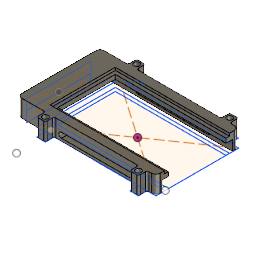
Mounting_plate_96_v3 v7 (Autodesk Fusion 360 design; units mm, degrees)
Autodesk Fusion 360 part; units mm, degrees
note: some values were not read from the file. Set by a fixed rule: which sketch regions a step uses.
sketch "Sketch1" plane through (0, 0, 0) normal (0, 0, 1) x (1, 0, 0)
  line L0 (-68.38, 47.37) -> (68.38, 47.37)
  line L1 (68.38, 47.37) -> (68.38, -47.37)
  line L2 (68.38, -47.37) -> (-68.38, -47.37)
  line L3 (-68.38, -47.37) -> (-68.38, 47.37)
  line L4 (-68.38, 47.37) -> (68.38, -47.37) construction
  line L5 (68.38, 47.37) -> (-68.38, -47.37) construction
  line L6 (-58.38, 57.37) -> (-48.38, 57.37)
  line L7 (-48.38, 57.37) -> (-48.38, 47.37)
  line L8 (-48.38, 47.37) -> (-58.38, 47.37)
  line L9 (-58.38, 47.37) -> (-58.38, 57.37)
  line L10 (48.38, 57.37) -> (58.38, 57.37)
  line L11 (58.38, 57.37) -> (58.38, 47.37)
  line L12 (58.38, 47.37) -> (48.38, 47.37)
  line L13 (48.38, 47.37) -> (48.38, 57.37)
  line L14 (48.38, -47.37) -> (58.38, -47.37)
  line L15 (58.38, -47.37) -> (58.38, -57.37)
  line L16 (58.38, -57.37) -> (48.38, -57.37)
  line L17 (48.38, -57.37) -> (48.38, -47.37)
  line L18 (-58.38, -47.37) -> (-48.38, -47.37)
  line L19 (-48.38, -47.37) -> (-48.38, -57.37)
  line L20 (-48.38, -57.37) -> (-58.38, -57.37)
  line L21 (-58.38, -57.37) -> (-58.38, -47.37)
  line L22 (68.38, 47.37) -> (68.38, 37)
  line L23 (68.38, -47.37) -> (68.38, -36.63)
  line L24 (68.38, 37) -> (-62.58, 37)
  line L25 (-62.58, 37) -> (-62.58, -37)
  line L26 (-62.58, -37) -> (68.38, -37)
  line L27 (68.38, -37) -> (68.38, 37)
  line L28 (68.38, 37) -> (68.38, 33)
  line L29 (68.38, 33) -> (-58.58, 33)
  line L30 (-58.58, 33) -> (-58.58, -33)
  line L31 (-58.58, -33) -> (68.38, -33)
  line L32 (68.38, -33) -> (68.38, 33)
  point P0 (-57.3369, -42.2056)
  point P1 (-53.88, -84.89)
  dimension "d1" = 136.76
  dimension "d2" = 94.74
  dimension "d3" = 10
  dimension "d4" = 10
  dimension "d5" = 10
  dimension "d6" = 10
  dimension "d15" = 10.37
  dimension "d16" = 10.74
  dimension "d17" = 74
  dimension "d18" = 130.96
  dimension "d19" = 4
  dimension "d20" = 66
  dimension "d21" = 126.96
  constraint perpendicular L0 L1
  constraint parallel L0 L2
  constraint parallel L1 L3
  constraint horizontal L0
  constraint horizontal L6
  constraint vertical L7
  constraint horizontal L8
  constraint vertical L9
  constraint coincident L0 L7.end
  constraint horizontal L10
  constraint vertical L11
  constraint horizontal L12
  constraint vertical L13
  constraint horizontal L14
  constraint vertical L15
  constraint horizontal L16
  constraint vertical L17
  constraint horizontal L18
  constraint vertical L19
  constraint horizontal L20
  constraint vertical L21
  constraint perpendicular L0 L22
  constraint perpendicular L2 L23
  constraint horizontal L24
  constraint vertical L25
  constraint horizontal L26
  constraint vertical L27
  constraint perpendicular L24 L28
  constraint horizontal L29
  constraint vertical L30
  constraint horizontal L31
  constraint vertical L32
  measures "d1" distance of L1 L3
  measures "d2" distance of L0.start L2.end
  measures "d3" distance of L6.start L6.end
  measures "d4" distance of L6.start L8.end
  measures "d5" distance of L10.start L10.end
  measures "d6" distance of L10.start L12.end
  measures "d15" distance of L0.end L22.end
  measures "d16" distance of L1.end L23.end
  measures "d17" distance of L22.end L26.end
  measures "d18" distance of L22.end L24.end
  measures "d19" distance of L22.end L28.end
  measures "d20" distance of L28.end L31.end
  measures "d21" distance of L28.end L29.end
  measures "d160" distance of L0.end
extrude "Extrude2" add sketch "Sketch1" along normal blind 20 contours L0 L1 L2 L3 L8 L12 L14 L18 L22 L23 L24 L25 L26 | L0 L6 L7 L8 L9 | L2 L18 L19 L20 L21 | L0 L10 L11 L12 L13 | L2 L14 L15 L16 L17 | L1 L23 L24 L25 L26 L27 L28 L29 L30 L31
ref_plane "WorkPlane2" through (0, 0, 20) normal (0, 0, 1) x (1, 0, 0)
sketch "Sketch4" plane through (0, 0, 20) normal (0, 0, 1) x (1, 0, 0)
  line L0 (68.38, 37) -> (-62.58, 37)
  line L1 (-62.58, 37) -> (-62.58, -37.7)
  line L2 (-62.58, -37.7) -> (68.38, -37.7)
  line L3 (68.38, -37.7) -> (68.38, 37)
  dimension "d30" = 130.96
  dimension "d31" = 74.7
  constraint horizontal L0
  constraint vertical L1
  constraint horizontal L2
  constraint vertical L3
  measures "d30" distance of L0.start L0.end
  measures "d31" distance of L0.start L2.end
extrude "Extrude3" cut sketch "Sketch4" against normal blind 3
ref_plane "WorkPlane3" through (0, 0, 20) normal (0, 0, 1) x (1, 0, 0)
sketch "Sketch5" plane through (0, 0, 20) normal (0, 0, 1) x (1, 0, 0)
  circle A0 centre (-53.38, 52.37) radius 3.25
  circle A1 centre (53.38, 52.37) radius 3.25
  circle A2 centre (-53.38, -52.37) radius 3.25
  circle A3 centre (53.38, -52.37) radius 3.25
  dimension "d35" = 6.5
  dimension "d38" = 106.76
  dimension "d39" = -104.74
  measures "d35" diameter of A0
extrude "Extrude4" cut sketch "Sketch5" against normal blind 20
ref_plane "WorkPlane5" through (68.38, 0, 0) normal (1, 0, 0) x (0, 1, 0)
ref_plane "WorkPlane6" through (68.38, 0, 0) normal (1, 0, 0) x (0, 1, 0)
sketch "Sketch7" plane through (68.38, 0, 0) normal (1, 0, 0) x (0, 1, 0)
  line L0 (40.5, 12) -> (-40.5, 12)
  line L1 (-40.5, 12) -> (-40.5, -12)
  line L2 (-40.5, -12) -> (40.5, -12)
  line L3 (40.5, -12) -> (40.5, 12)
  line L4 (40.5, 12) -> (-40.5, -12) construction
  line L5 (-40.5, 12) -> (40.5, -12) construction
  dimension "d45" = 81
  dimension "d46" = 24
  constraint perpendicular L0 L1
  constraint parallel L0 L2
  constraint parallel L1 L3
  constraint horizontal L0
  constraint coincident L4 origin
  constraint coincident L5 origin
  measures "d45" distance of L1.end L2.end
  measures "d46" distance of L0.end L1.end
extrude "Extrude5" cut sketch "Sketch7" against normal blind 136.76
fillet "Fillet2" radius 2 16 edges at (-58.38, 57.37, 10) (-58.38, 47.37, 10) (-58.38, -47.37, 10) (-58.38, -57.37, 10) (-48.38, -57.37, 10) (-48.38, -47.37, 10) (58.38, -57.37, 10) (58.38, -47.37, 10) (48.38, -47.37, 10) (48.38, -57.37, 10) (58.38, 47.37, 10) (58.38, 57.37, 10) (48.38, 47.37, 10) (48.38, 57.37, 10) (-48.38, 47.37, 10) (-48.38, 57.37, 10)
ref_plane "WorkPlane7" through (0, -47.37, 10) normal (0, -1, 0) x (1, 0, 0)
delete_face "DeleteFace1" 1 faces at (15.46, -47.37, 6.6667)
ref_plane "WorkPlane9" through (0, -47.37, 10) normal (0, -1, 0) x (1, 0, 0)
sketch "Sketch10" plane through (0, -47.37, 10) normal (0, -1, 0) x (1, 0, 0)
  line L0 (0, -10) -> (0, -4)
  line L1 (40, -7) -> (-40, -7)
  line L2 (-40, -7) -> (-40, -1)
  line L3 (-40, -1) -> (40, -1)
  line L4 (40, -1) -> (40, -7)
  line L5 (40, -7) -> (-40, -1) construction
  line L6 (-40, -7) -> (40, -1) construction
  circle A0 centre (-40, -4) radius 3
  circle A1 centre (40, -4) radius 3
  point P0 (0, -4)
  dimension "d72" = 6
  dimension "d73" = 6
  dimension "d74" = 80
  dimension "d75" = 6
  dimension "d76" = 6
  constraint vertical L0
  constraint perpendicular L1 L2
  constraint parallel L1 L3
  constraint parallel L2 L4
  constraint horizontal L1
  constraint coincident L5 P0
  constraint coincident L6 P0
  constraint coincident P0 L0.end
  constraint midpoint L2 A0.centre
  constraint midpoint L4 A1.centre
  measures "d72" distance of L0.start P0
  measures "d73" distance of L1.end L2.end
  measures "d74" distance of L2.end L3.end
  measures "d75" diameter of A0
  measures "d76" diameter of A1
extrude "Extrude9" cut sketch "Sketch10" against normal blind 6.87
ref_plane "WorkPlane10" through (0, 47.37, 10) normal (0, 1, 0) x (-1, 0, 0)
sketch "Sketch11" plane through (0, 47.37, 10) normal (0, 1, 0) x (1, 0, 0)
  line L0 (0, 10) -> (0, 4)
  line L1 (-40, 7) -> (40, 7)
  line L2 (40, 7) -> (40, 1)
  line L3 (40, 1) -> (-40, 1)
  line L4 (-40, 1) -> (-40, 7)
  line L5 (-40, 7) -> (40, 1) construction
  line L6 (40, 7) -> (-40, 1) construction
  circle A0 centre (40, 4) radius 3
  circle A1 centre (-40, 4) radius 3
  point P0 (0, 4)
  dimension "d80" = 6
  dimension "d81" = 80
  dimension "d82" = 6
  dimension "d83" = 6
  dimension "d84" = 6
  constraint vertical L0
  constraint perpendicular L1 L2
  constraint parallel L1 L3
  constraint parallel L2 L4
  constraint horizontal L1
  constraint coincident L5 P0
  constraint coincident L6 P0
  constraint coincident P0 L0.end
  constraint midpoint L2 A0.centre
  constraint midpoint L4 A1.centre
  measures "d80" distance of L0.start P0
  measures "d81" distance of L2.end L3.end
  measures "d82" distance of L1.end L2.end
  measures "d83" diameter of A0
  measures "d84" diameter of A1
extrude "Extrude10" cut sketch "Sketch11" against normal blind 6.87
ref_plane "WorkPlane11" through (0, 0, 0) normal (0, 0, 1) x (1, 0, 0)
sketch "Sketch12" plane through (0, 0, 0) normal (0, 0, 1) x (1, 0, 0)
ref_plane "WorkPlane12" through (-68.38, 0, 10) normal (-1, 0, 0) x (0, -1, 0)
ref_plane "WorkPlane13" through (-68.38, 0, 10) normal (-1, 0, 0) x (0, -1, 0)
sketch "Sketch19" plane through (68.38, 0, 0) normal (1, 0, 0) x (0, 1, 0)
ref_plane "WorkPlane19" through (-68.38, 0, 10) normal (-1, 0, 0) x (0, -1, 0)
sketch "Sketch21" plane through (-68.38, 0, 10) normal (-1, 0, 0) x (0, 1, 0)
  line L0 (42, -2) -> (-42, -2)
  line L1 (42, -2) -> (-42, 22) construction
  line L2 (-42, -2) -> (42, 22) construction
  line L3 (42, -2) -> (-42, -2)
  line L4 (-42, -2) -> (-42, 10)
  line L5 (-42, 10) -> (42, 10)
  line L6 (42, 10) -> (42, -2)
  point P0 (0, 10)
  dimension "d112" = 84
  dimension "d113" = 24
  constraint horizontal L0
  constraint coincident L1 P0
  constraint coincident L2 P0
  constraint horizontal L3
  constraint vertical L4
  constraint horizontal L5
  constraint vertical L6
  measures "d112" distance of L1.end L2.end
  measures "d113" distance of L0.end L1.end
ref_plane "WorkPlane25" through (-68.38, 0, 10) normal (-1, 0, 0) x (0, -1, 0)
sketch "Sketch27" plane through (-68.38, 0, 10) normal (-1, 0, 0) x (0, 1, 0)
  line L0 (-47.37, 30) -> (47.37, 30)
  line L1 (47.37, 30) -> (47.37, -10)
  line L2 (47.37, -10) -> (-47.37, -10)
  line L3 (-47.37, -10) -> (-47.37, 30)
  line L4 (-47.37, 30) -> (47.37, -10) construction
  line L5 (47.37, 30) -> (-47.37, -10) construction
  line L6 (47.37, 10) -> (-47.37, 10)
  point P0 (0, 10)
  dimension "d149" = 94.74
  dimension "d150" = 40
  constraint perpendicular L0 L1
  constraint parallel L0 L2
  constraint parallel L1 L3
  constraint horizontal L0
  constraint coincident L4 P0
  constraint coincident L5 P0
  constraint midpoint L1 L6.start
  constraint midpoint L3 L6.end
  measures "d149" distance of L1.end L2.end
  measures "d150" distance of L0.end L1.end
extrude "Extrude22" add sketch "Sketch27" along normal blind 22.07 contours L1 L2 L3 L6
ref_plane "WorkPlane26" through (-90.45, 0, 10) normal (-1, 0, 0) x (0, 0, 1)
sketch "Sketch28" plane through (-90.45, 0, 10) normal (-1, 0, 0) x (0, 1, 0)
  line L0 (-36.75, 22) -> (36.75, 22)
  line L1 (36.75, 22) -> (36.75, -2)
  line L2 (36.75, -2) -> (-36.75, -2)
  line L3 (-36.75, -2) -> (-36.75, 22)
  line L4 (-36.75, 22) -> (36.75, -2) construction
  line L5 (36.75, 22) -> (-36.75, -2) construction
  line L6 (36.75, 10) -> (-36.75, 10)
  point P0 (0, 10)
  dimension "d164" = 73.5
  dimension "d165" = 24
  constraint perpendicular L0 L1
  constraint parallel L0 L2
  constraint parallel L1 L3
  constraint horizontal L0
  constraint coincident L4 P0
  constraint coincident L5 P0
  constraint midpoint L1 L6.start
  constraint midpoint L3 L6.end
  measures "d164" distance of L1.end L2.end
  measures "d165" distance of L0.end L1.end
extrude "Extrude25" cut sketch "Sketch28" against normal blind 22.07 contours L1 L2 L3 L6
ref_plane "WorkPlane31" through (-68.38, 0, 10) normal (-1, 0, 0) x (0, 0, 1)
sketch "Sketch33" plane through (-68.38, 0, 10) normal (-1, 0, 0) x (0, 1, 0)
  line L0 (40.5, 22) -> (-40.5, 22)
  line L1 (-40.5, 22) -> (-40.5, -2)
  line L2 (-40.5, -2) -> (40.5, -2)
  line L3 (40.5, -2) -> (40.5, 22)
  line L4 (40.5, 22) -> (-40.5, -2) construction
  line L5 (-40.5, 22) -> (40.5, -2) construction
  point P0 (0, 10)
  dimension "d173" = 81
  dimension "d174" = 24
  constraint perpendicular L0 L1
  constraint parallel L0 L2
  constraint parallel L1 L3
  constraint horizontal L0
  constraint coincident L4 P0
  constraint coincident L5 P0
  measures "d173" distance of L1.end L2.end
  measures "d174" distance of L0.end L1.end
extrude "Extrude26" cut sketch "Sketch33" along normal blind 15.2
ref_plane "WorkPlane32" through (-11.035, 0, 12) normal (0, 0, -1) x (0, -1, 0)
fillet "Fillet6" radius 5 4 edges at (-90.45, 47.37, 10) (-90.45, -47.37, 10) (68.38, -47.37, 10) (68.38, 47.37, 10)
sketch "Sketch34" plane through (-11.035, 0, 12) normal (0, 0, -1) x (1, 0, 0)
  line L0 (-72.545, -36.75) -> (-86.285, -36.75)
  line L1 (-86.285, -36.75) -> (-86.285, 36.75)
  line L2 (-86.285, 36.75) -> (-72.545, 36.75)
  line L3 (-72.545, 36.75) -> (-72.545, -36.75)
  line L4 (-72.545, -36.75) -> (-86.285, 36.75) construction
  line L5 (-86.285, -36.75) -> (-72.545, 36.75) construction
  point P0 (-79.415, 0)
  dimension "d178" = 13.74
  dimension "d179" = 73.5
  constraint perpendicular L0 L1
  constraint parallel L0 L2
  constraint parallel L1 L3
  constraint horizontal L0
  constraint coincident L4 P0
  constraint coincident L5 P0
  measures "d178" distance of L1.end L2.end
  measures "d179" distance of L0.end L1.end
extrude "Extrude27" [suppressed]
ref_plane "WorkPlane27" through (-68.38, 0, 0) normal (1, 0, 0) x (0, 1, 0)
sketch "Sketch29" plane through (-68.38, 0, 0) normal (1, 0, 0) x (0, 1, 0)
  line L0 (40.5, 12) -> (-40.5, 12)
  line L1 (-40.5, 12) -> (-40.5, -12)
  line L2 (-40.5, -12) -> (40.5, -12)
  line L3 (40.5, -12) -> (40.5, 12)
  line L4 (40.5, 12) -> (-40.5, -12) construction
  line L5 (-40.5, 12) -> (40.5, -12) construction
  dimension "d159" = 24
  dimension "d160" = 81
  constraint perpendicular L0 L1
  constraint parallel L0 L2
  constraint parallel L1 L3
  constraint horizontal L0
  constraint coincident L4 origin
  constraint coincident L5 origin
  measures "d159" distance of L0.end L1.end
  measures "d160" distance of L1.end L2.end
extrude "Extrude24" [suppressed]
ref_plane "WorkPlane28" through (-11.035, 0, 12) normal (0, 0, -1) x (0, -1, 0)
sketch "Sketch30" plane through (-11.035, 0, 12) normal (0, 0, -1) x (1, 0, 0)
extrude "Extrude15" [suppressed]
ref_plane "WorkPlane20" through (-68.32, 0, 0) normal (1, 0, 0) x (0, 1, 0)
sketch "Sketch22" plane through (-68.32, 0, 0) normal (1, 0, 0) x (0, 1, 0)
  line L0 (40.5, -12) -> (-40.5, -12)
  line L1 (-40.5, -12) -> (-40.5, 12)
  line L2 (-40.5, 12) -> (40.5, 12)
  line L3 (40.5, 12) -> (40.5, -12)
  line L4 (40.5, -12) -> (-40.5, 12) construction
  line L5 (-40.5, -12) -> (40.5, 12) construction
  dimension "d117" = 81
  dimension "d118" = 24
  constraint perpendicular L0 L1
  constraint parallel L0 L2
  constraint parallel L1 L3
  constraint horizontal L0
  constraint coincident L4 origin
  constraint coincident L5 origin
  measures "d117" distance of L1.end L2.end
  measures "d118" distance of L0.end L1.end
extrude "Extrude16" [suppressed]
ref_plane "WorkPlane23" through (-76.98, 0, 12) normal (0, 0, 1) x (0, 1, 0)
sketch "Sketch25" plane through (-76.98, 0, 12) normal (0, 0, 1) x (1, 0, 0)
  line L0 (8.6, 42) -> (-8.6, 42)
  line L1 (-8.6, 42) -> (-8.6, -42)
  line L2 (-8.6, -42) -> (8.6, -42)
  line L3 (8.6, -42) -> (8.6, 42)
  dimension "d136" = 17.2
  dimension "d137" = 84
  constraint horizontal L0
  constraint vertical L1
  constraint horizontal L2
  constraint vertical L3
  measures "d136" distance of L0.start L0.end
  measures "d137" distance of L0.start L2.end
extrude "Extrude19" [suppressed]
fillet "Fillet5" [suppressed]
ref_plane "WorkPlane24" through (-85.58, 0, 6.5) normal (-1, 0, 0) x (0, -1, 0)
sketch "Sketch26" plane through (-85.58, 0, 6.5) normal (-1, 0, 0) x (0, 1, 0)
  line L0 (38, 18.5) -> (-38, 18.5)
  line L1 (-38, 18.5) -> (-38, -3.5)
  line L2 (-38, -3.5) -> (38, -3.5)
  line L3 (38, -3.5) -> (38, 18.5)
  line L4 (38, 18.5) -> (-38, -3.5) construction
  line L5 (-38, 18.5) -> (38, -3.5) construction
  point P0 (0, 7.5)
  dimension "d142" = 76
  dimension "d143" = 22
  constraint perpendicular L0 L1
  constraint parallel L0 L2
  constraint parallel L1 L3
  constraint horizontal L0
  constraint coincident L4 P0
  constraint coincident L5 P0
  measures "d142" distance of L1.end L2.end
  measures "d143" distance of L0.end L1.end
extrude "Extrude21" [suppressed]
extrude "Extrude20" [suppressed]
fillet "Fillet3" [suppressed]
fillet "Fillet4" [suppressed]
ref_plane "WorkPlane21" through (-85.58, 0, 5) normal (-1, 0, 0) x (0, 0, 1)
ref_plane "WorkPlane22" through (-85.58, 0, 5) normal (-1, 0, 0) x (0, 0, 1)
sketch "Sketch24" plane through (-85.58, 0, 5) normal (-1, 0, 0) x (0, 1, 0)
  line L0 (-38, 11) -> (38, 11)
  line L1 (38, 11) -> (38, -3)
  line L2 (38, -3) -> (-38, -3)
  line L3 (-38, -3) -> (-38, 11)
  line L4 (-38, 11) -> (38, -3) construction
  line L5 (38, 11) -> (-38, -3) construction
  point P0 (0, 4)
  dimension "d131" = 76
  dimension "d132" = 14
  constraint perpendicular L0 L1
  constraint parallel L0 L2
  constraint parallel L1 L3
  constraint horizontal L0
  constraint coincident L4 P0
  constraint coincident L5 P0
  measures "d131" distance of L1.end L2.end
  measures "d132" distance of L0.end L1.end
extrude "Extrude18" [suppressed]
